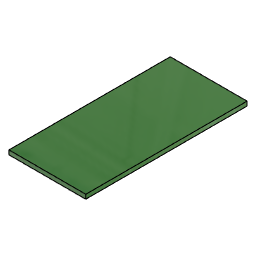
estrucutra v3 (Autodesk Fusion 360 archive; units mm, degrees)
design "taulellç"
Autodesk Fusion 360 part; units mm, degrees
sketch "Boceto1" plane through (0, 0, 0) normal (0, 0, 1) x (1, 0, 0)
  line L0 (0, 500) -> (450, 500)
  line L1 (450, 500) -> (450, -445)
  line L2 (450, -445) -> (0, -445)
  line L3 (0, -445) -> (0, 500)
  dimension "d1" = 450
  dimension "d2" = 945
  constraint horizontal L0
  constraint vertical L1
  constraint horizontal L2
  constraint vertical L3
  measures "d1" distance of L0.start L0.end
  measures "d2" distance of L0.start L2.end
extrude "Extruir1" add sketch "Boceto1" along normal blind 25

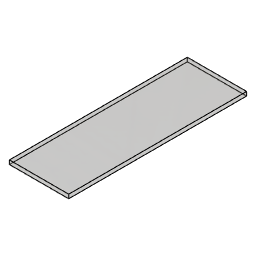
design "metracilat pantalla"
Autodesk Fusion 360 part; units mm, degrees
sketch "Boceto1" plane through (0, 0, 0) normal (0, 0, 1) x (1, 0, 0)
  line L0 (0, 0) -> (150, 0)
  line L1 (150, 0) -> (150, 450)
  line L2 (150, 450) -> (0, 450)
  line L3 (0, 450) -> (0, 0)
  dimension "d1" = 150
  dimension "d2" = 450
  constraint horizontal L0
  constraint vertical L1
  constraint horizontal L2
  constraint vertical L3
  constraint coincident L0.start L3.end
  measures "d1" distance of L0.start L0.end
  measures "d2" distance of L0.start L2.end
extrude "Extruir1" add sketch "Boceto1" along normal blind 10

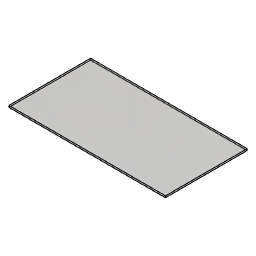
design "metracilat joc"
Autodesk Fusion 360 part; units mm, degrees
sketch "Boceto1" plane through (0, 0, 0) normal (0, 0, 1) x (1, 0, 0)
  line L0 (963.8754, 9.656) -> (5.8754, 9.656)
  line L1 (5.8754, 9.656) -> (5.8754, 509.656)
  line L2 (5.8754, 509.656) -> (963.8754, 509.656)
  line L3 (963.8754, 509.656) -> (963.8754, 9.656)
  dimension "d1" = 958
  dimension "d2" = 500
  constraint horizontal L0
  constraint vertical L1
  constraint horizontal L2
  constraint vertical L3
  measures "d1" distance of L0.start L0.end
  measures "d2" distance of L0.start L2.end
extrude "Extruir1" add sketch "Boceto1" along normal blind 10
